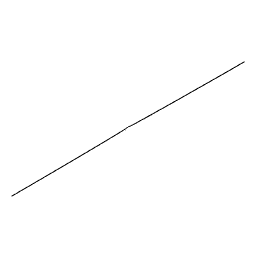
Segment porteur BZ suspension (communication) (Autodesk Fusion 360 design; units mm, degrees)
Autodesk Fusion 360 part; units mm, degrees
sketch "Sketch1" plane through (0, 0, 0) normal (1, 0, 0) x (0, 0, -1)
  arc A0 (-27.7506, 37.9459) -> (-69.985, 34.9963) centre (0, -663.2552) ccw construction
  arc A1 (12.25, 38.3879) -> (-12.2506, 38.3879) centre (0, -663.2552) ccw construction
  arc A2 (69.985, 34.9963) -> (27.75, 37.9459) centre (0, -663.2552) ccw construction
  arc A3 (69.985, 34.9963) -> (-69.985, 34.9963) centre (0, -663.2552) ccw
  line L0 (0, 0) -> (0, 500) construction
  line L1 (45000, 0) -> (45000, 500) construction
  line L2 (0, 0) -> (45000, 0) construction
  line L3 (0, -1000) -> (45000, -1000) construction
  line L4 (22500, -1000) -> (22500, 860) construction
  line L5 (69.985, 34.9963) -> (652.2509, -23.3635)
  line L6 (22500, -1000) -> (20189.199, -1000)
  arc A4 (652.2509, -23.3635) -> (20189.199, -1000) centre (20189.199, 194900) ccw
  arc A5 (-20189.199, -1000) -> (-652.2509, -23.3635) centre (-20189.199, 194900) ccw
  line L7 (-652.2509, -23.3635) -> (-69.985, 34.9963)
  dimension "d3" = 500
  dimension "d51" = 45000
  dimension "d52" = 1000
  dimension "d53" = 195900
  constraint coincident A0.end A3.end
  constraint coincident L0.start L2.start
  constraint perpendicular L1 L2
  constraint midpoint L3 L4.start
  constraint perpendicular L2 L4
  constraint coincident A2.start A3.start
  constraint tangent A2 L5
  constraint perpendicular L4 L6
  constraint tangent L6 A4
  constraint tangent L5 A4
  constraint symmetric L0 L6.end A5.start
  constraint symmetric L0 L5.end A5.end
  constraint symmetric L0 A4 A5
  constraint tangent A3 L7
  measures "d3" distance of L0.start L0.end
  measures "d53" radius of A4
sketch "Sketch2" plane through (0, 0, 0) normal (0, 0, 1) x (1, 0, 0)
  line L0 (0, 34.9963) -> (0, 38.4948) construction
  circle A0 centre (0, 44.5698) radius 6.075
  dimension "d6" = 12.15
  constraint coincident L0.end A0
  measures "d6" diameter of A0
sweep "Sweep1" add profiles "Sketch2" path "Sketch1" along A5 L7 A3 L5 A4 L6 section 1 makes body 1
sketch "Sketch3" plane through (0, 0, 0) normal (1, 0, 0) x (0, 0, -1)
  line L0 (69.985, 34.9963) -> (71.1967, 47.0857) construction
  line L1 (-71.1967, 47.0857) -> (-69.985, 34.9963) construction
  arc A0 (69.985, 34.9963) -> (-69.985, 34.9963) centre (0, -663.2552) ccw construction
  line L2 (-69.985, 34.9963) -> (-69.985, 31.0963) construction
  line L3 (69.985, 34.9963) -> (69.985, 31.0963) construction
  arc A1 (69.985, 31.0963) -> (-69.985, 31.0963) centre (0, -296.2107) ccw
  line L4 (0, 0) -> (0, 140) construction
  line L5 (22500, 0) -> (22500, 140) construction
  line L6 (22500, 0) -> (0, 0) construction
  line L7 (0, 38.4948) -> (22500, 38.4948) construction
  line L8 (0, 38.4948) -> (0, -600)
  line L9 (4500, 38.4948) -> (4500, -600) construction
  line L10 (11250, 38.4948) -> (11250, -600) construction
  line L11 (18000, 38.4948) -> (18000, -600) construction
  line L12 (4500, -151.5052) -> (5900, 2000) construction
  line L13 (11250, 38.4948) -> (11250, -241.5052) construction
  line L14 (11250, -241.5052) -> (12029.611, 752.3193)
  line L15 (18000, 38.4948) -> (18000, -291.5052) construction
  line L16 (18000, -291.5052) -> (19200, 1100)
  line L17 (22500, 38.4948) -> (22500, -301.5052) construction
  line L18 (22500, -301.5052) -> (24000, 1200) construction
  spline S0 degree 5 poles (22500, -301.5052) (22355.8041, -301.7386) (22062.2297, -302.0887) (21606.3204, -302.2641) (20967.2636, -301.7964) (20116.5315, -300.0372) (19214.8524, -297.106) (18264.844, -293.0228) (17271.4075, -287.8334) (16242.745, -281.6235) (15189.3924, -274.5033) (14122.5824, -266.582) (13052.8924, -257.9476) (11988.6891, -248.6423) (10934.8488, -238.6433) (9890.8283, -227.8335) (8850.5629, -216.0007) (7806.8474, -202.9063) (6754.8867, -188.3426) (5696.0714, -172.1914) (4641.9917, -154.4929) (3617.806, -135.4897) (2667.7426, -115.7442) (1841.7386, -95.5944) (1178.7692, -74.4839) (691.844, -50.3668) (418.8243, -25.2579) (240.6163, -0.038) (126.1424, 20.1548) (69.985, 31.0963) knots 0 0 0 0 0 0 0.04 0.08 0.12 0.16 0.2 0.24 0.28 0.32 0.36 0.4 0.44 0.48 0.52 0.56 0.6 0.64 0.68 0.72 0.76 0.8 0.84 0.88 0.92 0.96 1 1 1 1 1 1
  line L19 (1993.3183, -343.6376) -> (-1853.3484, 405.8302)
  point P0 (-27.7506, 37.9459)
  point P1 (12.25, 38.3879)
  point P2 (-12.2506, 38.3879)
  point P3 (27.75, 37.9459)
  point P4 (750, -50)
  dimension "d55" = 3.9
  dimension "d56" = 3.9
  dimension "d57" = 22500
  dimension "d59" = 4500
  dimension "d60" = 11250
  dimension "d61" = 18000
  dimension "d62" = 190
  dimension "d63" = 280
  dimension "d64" = 330
  dimension "d65" = 340
  constraint coincident L1.end A0.end
  constraint coincident L0.start A0.start
  constraint tangent A0 A1
  constraint coincident L4.start L6.end
  constraint vertical L4
  constraint perpendicular L4 L6
  constraint midpoint A0 L7.start
  constraint tangent A0 L7
  constraint coincident L5 L7.end
  constraint perpendicular L7 L8
  constraint midpoint L3.end L19
  measures "d55" distance of L1.end L2.end
  measures "d56" distance of L0.start L3.end
  measures "d62" distance of L9.start L12.start
  measures "d63" distance of L10.start L13.end
  measures "d64" distance of L11.start L15.end
  measures "d65" distance of L7.end L17.end
sweep "Sweep2" add profiles "Sketch2" path "Sketch3" along S0 A1 section 1 separate body makes body 2
mirror "Mirror1" about plane through (0, 0, 0) normal (0, 0, 1) of bodies 2 makes body 3
hidden bodies 1
equation "d51 = 4.500E+04 mm"
equation "d53 = 1.959E+05 mm"
equation "d57 = 2.250E+04 mm"
equation "d60 = 1.125E+04 mm"
equation "d61 = 1.800E+04 mm"
named bodies: "Body1 - Old", "Body2 - New", "Body2 - New (1)"
